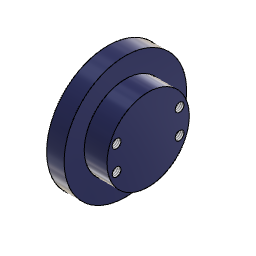
Encaixe Segurador da Garra v6 (Autodesk Fusion 360 design; units mm, degrees)
Autodesk Fusion 360 part; units mm, degrees
sketch "Sketch1" plane through (0, 0, 0) normal (1, 0, 0) x (0, 1, 0)
  circle A0 centre (0, 0) radius 35
  dimension "d1" = 70
  constraint coincident A0.centre origin
  measures "d1" diameter of A0
extrude "Extrude1" add sketch "Sketch1" along normal blind 10 in component "Encaixe"
sketch "Sketch3" plane through (10, 0, 0) normal (1, 0, 0) x (0, 1, 0)
  circle A0 centre (0, 0) radius 35
  circle A1 centre (0, 0) radius 23.5
  dimension "d9" = 47
  constraint coincident A0.centre A1.centre
  measures "d9" diameter of A1
extrude "Extrude2" add sketch "Sketch3" along normal blind 13 contours A1 in component "Encaixe"
ref_plane "WorkPlane1" through (0, 13, 0) normal (0, 1, 0) x (0, 0, 1)
sketch "Sketch4" plane through (0, 13, 0) normal (0, 1, 0) x (1, 0, 0)
  line L0 (23, 0) -> (23, -35)
  line L1 (23, -35) -> (23, -45)
  line L2 (23, -35) -> (30.3921, -43.8095)
  line L3 (30.3921, -43.8095) -> (35.3921, -43.8095)
  line L4 (23, 0) -> (57, 0)
  line L5 (35.3921, -43.8095) -> (52.4338, -23.5)
  line L6 (35.3921, -43.8095) -> (44, -43.8095)
  line L7 (52.4338, -23.5) -> (52.4338, 0)
  line L8 (52.4338, 23.5) -> (52.4338, 0)
  line L9 (35.3921, 43.8095) -> (52.4338, 23.5)
  line L10 (30.3921, 43.8095) -> (35.3921, 43.8095)
  line L11 (23, 35) -> (30.3921, 43.8095)
  line L12 (23, 0) -> (23, 35)
  dimension "d13" = 35
  dimension "d14" = 10
  dimension "d15" = 11.5
  dimension "d16" = 40
  dimension "d17" = 5
  dimension "d18" = 50
  constraint vertical L0
  constraint parallel L0 L1
  constraint horizontal L3
  constraint perpendicular L0 L4
  constraint parallel L3 L6
  constraint coincident L4 L7.end
  constraint perpendicular L4 L7
  constraint symmetric L0.start L4 L12.start
  constraint symmetric L0.end L4 L11.start
  constraint symmetric L2.end L4 L10.start
  constraint symmetric L3.end L4 L9.start
  constraint symmetric L4 L5.end L8.start
  constraint symmetric L4 L7.end L8.end
  measures "d13" distance of L0.start L0.end
  measures "d14" distance of L0.end L1.end
  measures "d15" distance of L0.end L2.end
  measures "d16" angle of L1 L2
  measures "d17" distance of L2.end L3.end
  measures "d18" angle of L5 L6
sketch "Sketch10" plane through (23, 0, 0) normal (1, 0, 0) x (0, 1, 0)
  circle A0 centre (0, 0) radius 23.5
  line L0 (0, 0) -> (18.3161, -14.7232) construction
  line L1 (0, 0) -> (18.3161, 14.7232) construction
  line L2 (0, 0) -> (-18.3161, 14.7232) construction
  line L3 (0, 0) -> (-18.3161, -14.7232) construction
  arc A1 (18.3161, -14.7232) -> (18.3161, 14.7232) centre (0, 0) ccw construction
  arc A2 (-18.3161, 14.7232) -> (-18.3161, -14.7232) centre (0, 0) ccw construction
  line L4 (0, 0) -> (-23.5, 0) construction
  line L5 (-23.5, 0) -> (-18, 0)
  line L6 (-18, 0) -> (-18, 7) construction
  circle A3 centre (-18, 7) radius 3
  circle A4 centre (-18, -7) radius 3
  line L7 (0, 0) -> (0, 10) construction
  circle A5 centre (18, 7) radius 3
  circle A6 centre (18, -7) radius 3
  dimension "d43" = 102.413
  dimension "d45" = 6
  constraint coincident A0.centre L0.start
  constraint coincident A0 L0.end
  constraint coincident A0 L1.end
  constraint coincident A0 L2.end
  constraint parallel L0 L2
  constraint coincident A0 L3.end
  constraint parallel L1 L3
  constraint equal A1 A2
  constraint midpoint A2 L4.end
  constraint horizontal L4
  constraint coincident L4 L5.end
  constraint perpendicular L4 L6
  constraint coincident L6.end A3.centre
  constraint symmetric L4 A3 A4
  constraint vertical L7
  constraint symmetric A3 L7 A5
  constraint symmetric A4 L7 A6
  measures "d43" angle of L1 L2
  measures "d45" diameter of A3
extrude "Extrude8" cut sketch "Sketch10" against normal blind 10 contours A3 | A4 | A5 | A6 in component "Encaixe"
thread "Thread1" "ISO Metric profile 6.0 M6x1 6H" major diameter 6.147 minor diameter 5.035 pitch 1 angle 60 resizes the face on face at (16.3333, -15.0037, 6.8505) in component "Encaixe"
thread "Thread2" "ISO Metric profile 6.0 M6x1 6H" major diameter 6.147 minor diameter 5.035 pitch 1 angle 60 resizes the face on face at (16.3333, 20.9963, 6.8505) in component "Encaixe"
thread "Thread3" "ISO Metric profile 6.0 M6x1 6H" major diameter 6.147 minor diameter 5.035 pitch 1 angle 60 resizes the face on face at (16.3333, -15.0037, -7.1495) in component "Encaixe"
thread "Thread4" "ISO Metric profile 6.0 M6x1 6H" major diameter 6.147 minor diameter 5.035 pitch 1 angle 60 resizes the face on face at (16.3333, 20.9963, -7.1495) in component "Encaixe"
sketch "Sketch11" plane through (0, 0, 0) normal (-1, 0, 0) x (0, -1, 0)
  circle A0 centre (0, 0) radius 35
  circle A1 centre (0, 0) radius 10
  dimension "d48" = 20
  constraint concentric A0 A1
  measures "d48" diameter of A1
extrude "Extrude9" cut sketch "Sketch11" against normal blind 10 contours A1 in component "Encaixe"
extrude "Extrude10" cut 1 faces at (10, -3.1852, -0.9825) along direction (1, 0, 0) blind 5 in component "Encaixe"
sketch "Sketch12" plane through (15, 0, 0) normal (-1, 0, 0) x (0, -1, 0)
  circle A0 centre (0, 0) radius 10
  line L0 (3, 3) -> (3, 9.5394)
  line L1 (-3, 3) -> (-3, 9.5394)
  line L2 (-3, -3) -> (-9.5394, -3)
  line L3 (-3, 3) -> (-9.5394, 3)
  line L4 (3, -3) -> (3, -9.5394)
  line L5 (-3, -3) -> (-3, -9.5394)
  line L6 (3, 3) -> (9.5394, 3)
  line L7 (3, -3) -> (9.5394, -3)
  constraint coincident A0 L0.end
  constraint coincident A0 L1.end
  constraint coincident A0 L3.end
  constraint coincident A0 L2.end
  constraint coincident A0 L6.end
  constraint coincident A0 L7.end
  constraint coincident A0 L4.end
  constraint coincident A0 L5.end
extrude "Extrude11" add sketch "Sketch12" along normal blind 15 contours A0 L0 L6 | A0 L4 L7 | A0 L1 L3 | A0 L2 L5 in component "Encaixe"
component "Encaixe" placed x (1, 0, 0) y (0, 1, 0) z (0, 0, 1) at (0, 0, 0)
